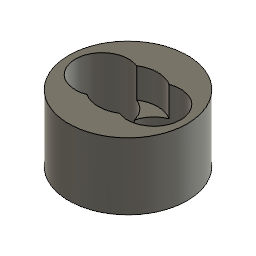
as5600 磁铁放置 (Autodesk Fusion 360 design; units mm, degrees)
part number: 2026-08-19-09-30-43-938
Autodesk Fusion 360 part; units mm, degrees
sketch "草图1" plane through (0, 0, 0) normal (0, 1, 0) x (1, 0, 0)
  circle A0 centre (0, 0) radius 4
  dimension "d1" = 8
  constraint coincident A0.centre origin
  measures "d1" diameter of A0
extrude "拉伸1" add sketch "草图1" along normal blind 4.5
sketch "草图2" plane through (0, 4.5, 0) normal (0, 1, 0) x (-1, 0, 0)
  circle A0 centre (0, 0) radius 4
  circle A1 centre (0, 0) radius 2
  dimension "d4" = 4
  constraint concentric A0 A1
  measures "d4" diameter of A1
extrude "拉伸2" cut sketch "草图2" against normal blind 2 contours A1
sketch "草图3" plane through (0, 4.5, 0) normal (0, 1, 0) x (-1, 0, 0)
  circle A0 centre (0, 0) radius 2
  circle A1 centre (0, 0) radius 4
  circle A2 centre (1.75, 0) radius 1.8
  circle A3 centre (-1.75, 0) radius 1.8
  dimension "d7" = 3.6
  dimension "d8" = 3.6
  dimension "d9" = 3.5
  measures "d7" diameter of A2
  measures "d8" diameter of A3
  measures "d9" distance of A2.centre A3.centre
extrude "拉伸3" cut sketch "草图3" against normal blind 3.7 contours A0 A2 A3 | A0 A2 | A0 A2 A3 | A0 A3 | A2 A3 picked at (0.6739, -0.4996) picked at (-0.6772, -0.4762)
sketch "草图4" plane through (0, 4.5, 0) normal (0, 1, 0) x (-1, 0, 0)
  circle A0 centre (1.75, 0) radius 1
  circle A1 centre (-1.75, 0) radius 1
  dimension "d12" = 2
  dimension "d13" = 2
  measures "d12" diameter of A0
  measures "d13" diameter of A1
extrude "拉伸4" cut sketch "草图4" against normal blind 4.5
